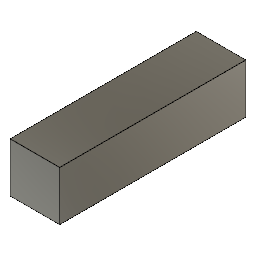
HeleShawVideoApparatus-ShortPillar v4 (Autodesk Fusion 360 design; units mm, degrees)
Autodesk Fusion 360 part; units mm, degrees
sketch "Sketch1" plane through (0, 0, 0) normal (0, 0, 1) x (1, 0, 0)
  line L0 (10, -45) -> (-10, -45)
  line L1 (-10, -45) -> (-10, 45)
  line L2 (-10, 45) -> (10, 45)
  line L3 (10, 45) -> (10, -45)
  line L4 (10, -45) -> (-10, 45) construction
  line L5 (-10, -45) -> (10, 45) construction
  dimension "d1" = 20
  dimension "d2" = 90
  constraint perpendicular L0 L1
  constraint parallel L0 L2
  constraint parallel L1 L3
  constraint horizontal L0
  constraint coincident L4 origin
  constraint coincident L5 origin
  measures "d1" distance of L1.end L2.end
  measures "d2" distance of L0.end L1.end
extrude "Extrude1" add sketch "Sketch1" along normal blind 20
extrude "Extrude2" add 1 faces at (-3.3333, 45, 6.6667) along direction (0, 1, 0) blind 10
extrude "Extrude3" cut 1 faces at (3.3333, -45, 6.6667) along direction (0, 1, 0) blind 39.2
extrude "Extrude4" add 1 faces at (3.3333, -5.8, 6.6667) along direction (0, -1, 0) blind 14.2
